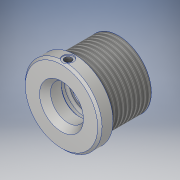
# Autodesk Inventor part: reservoir_jointure
Saved by Autodesk Inventor 2019 (Build 230136000, 136)
## iProperties
Created: 2019-03-25
Part Number: reservoir_jointure
Material: Aluminium 6061
Document SubType Name: Modeling
Designer: theor
Density: 2.7 g/cm^3
Appearance: Aluminium - Plat
Mass: 63.5199 g
Surface Area: 90.4788 cm^2
Volume: 23.5259 cm^3
Author: theor
Autodesk Inventor part; units mm, degrees
ref_plane "YZ Plane" through (0, 0, 0) normal (1, 0, 0) x (0, 1, 0)
ref_plane "XY Plane" through (0, 0, 0) normal (0, 0, 1) x (1, 0, 0)
sketch "Esquisse1" plane through (0, 0, 0) normal (1, 0, 0) x (0, 1, 0)
  line L0 (0, 0) -> (0, -31.3963)
  line L1 (8, -3) -> (8, -8.5)
  line L2 (16.5, 0) -> (10, 0)
  line L3 (10, 0) -> (8, -3)
  circle A0 centre (8, -10) radius 1.5 construction
  line L4 (8, -8.5) -> (9.5, -8.5)
  line L5 (9.5, -8.5) -> (9.5, -11.9749)
  line L6 (9.5, -11.9749) -> (6, -11)
  line L7 (6, -11) -> (6, -16)
  line L8 (6, -16) -> (14, -26)
  line L9 (14, -26) -> (15, -26)
  line L10 (15, -26) -> (15, -6)
  line L11 (15, -6) -> (17.5, -6)
  line L12 (17.5, -6) -> (17.5, -1)
  line L13 (16.5, 0) -> (17.5, -1)
  dimension "d3" = 16
  dimension "d4" = 3
  dimension "d5" = 2
  dimension "d7" = 3
  dimension "d9" = 12
  dimension "d10" = 2.5
  dimension "d11" = 11
  dimension "d12" = 5
  dimension "d13" = 1
  dimension "d14" = 30
  dimension "d15" = 10
  dimension "d19" = 2.5
  dimension "d20" = 20
  dimension "d97" = 1
  dimension "d98" = 1
  constraints: 28 end point, 6 vertical, 4 horizontal, 3 tangent, 1 centre point, 1 horizontal alignment, 1 vertical alignment
  measures "d3" diameter of L1 L0
  measures "d4" vertical distance of L2.end L1.start
  measures "d5" horizontal distance of L2.end L1.start
  measures "d7" diameter of A0
  measures "d9" diameter of L7 L0
  measures "d10" vertical distance of L1.end L6.end
  measures "d11" vertical distance of L2.end L6.end
  measures "d12" distance of L6.end L7.end
  measures "d13" distance of L8.end L9.end
  measures "d14" diameter of L9.end L0
  measures "d15" vertical distance of L7.end L8.end
  measures "d19" distance of L10.end L11.end
  measures "d20" distance of L9.end L10.end
  measures "d97" horizontal distance of L2.start L12.end
  measures "d98" horizontal distance of L2.start L12.end
revolve "Révolution1" add sketch "Esquisse1" angle 360 about axis through (0, 0, 0) along (0, 0, -1)
thread "Filetage1" size "M30x2" class "6g" standard "ISO Metric profile" full length
fillet "Congé1" radius 1 1 edges at (0, -9.5, -11.9749)
chamfer "Chanfrein1" distance 0.5 angle 45 3 edges at (0, -8, -8.5) (0, -6, -11) (0, -9.5, -8.5)
ref_plane "Plan de construction3" through (0, 17.5, -3.5) normal (0, 1, 0) x (-1, 0, 0)
sketch "Esquisse9" plane through (0, 17.5, -3.5) normal (0, 1, 0) x (-1, 0, 0)
  circle A0 centre (0, 0.5) radius 2.5
  line L0 (-10, 3.5) -> (10, 3.5) projected
  line L1 (-8, 0.5) -> (8, 0.5) projected
  point P0 (0, 3.5)
  point P1 (0, 3.5)
  dimension "d85" = 5
  constraints: 2 midpoint, 1 centre point, 1 coincident, 1 vertical alignment
  measures "d85" diameter of A0
extrude "Extrusion4" cut sketch "Esquisse9" against normal blind 0.5
sketch "Esquisse10" plane through (0, 17, -3) normal (0, 1, 0) x (1, 0, 0)
  circle A0 centre (0, 0) radius 2.5 projected
  point P0 (0, -3)
  point P1 (0, -2.5)
  constraints: 1 coincident, 1 vertical alignment
hole "Perçage3" at (0, 17, -3) direction (0, -1, 0) diameter 3.242 depth 5.5 tip angle 118 thread size "M4x0.7" class "6H" standard "ISO Metric profile"
